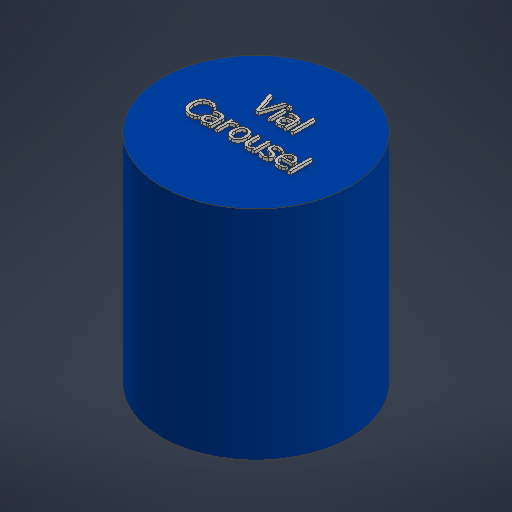
# Autodesk Inventor part: VialCarousel
Saved by Autodesk Inventor 2025.1 (Build 291241000, 241)
## iProperties
Created: 2024-10-04
Part Number: VialCarousel
Material: Generic
Document SubType Name: Modeling
Designer: jerem
Density: 1 g/cm^3
Appearance: Default
Author: jerem
Autodesk Inventor part; units mm, degrees
ref_plane "YZ Plane" through (0, 0, 0) normal (1, 0, 0) x (0, 1, 0)
ref_plane "XZ Plane" through (0, 0, 0) normal (0, 1, 0) x (-1, 0, 0)
ref_plane "XY Plane" through (0, 0, 0) normal (0, 0, 1) x (1, 0, 0)
sketch "Sketch1" plane through (0, 0, 0) normal (0, 1, 0) x (-1, 0, 0)
  circle A0 centre (0, 0) radius 65
  line L0 (0, 0) -> (0, -25) construction
  circle A1 centre (0, -25) radius 11.5 construction
  circle A2 centre (21.6506, -12.5) radius 11.5 construction
  circle A3 centre (21.6506, 12.5) radius 11.5 construction
  circle A4 centre (0, 25) radius 11.5 construction
  circle A5 centre (-21.6506, 12.5) radius 11.5 construction
  circle A6 centre (-21.6506, -12.5) radius 11.5 construction
  line L1 (0, 0) -> (-21.6506, 37.5) construction
  circle A7 centre (-21.6506, 37.5) radius 11.5 construction
  circle A8 centre (-43.3013, 0) radius 11.5 construction
  circle A9 centre (-21.6506, -37.5) radius 11.5 construction
  circle A10 centre (21.6506, -37.5) radius 11.5 construction
  circle A11 centre (43.3013, 0) radius 11.5 construction
  circle A12 centre (21.6506, 37.5) radius 11.5 construction
  circle A13 centre (0, 50) radius 11.5 construction
  circle A14 centre (-43.3013, 25) radius 11.5 construction
  circle A15 centre (-43.3013, -25) radius 11.5 construction
  circle A16 centre (0, -50) radius 11.5 construction
  circle A17 centre (43.3013, -25) radius 11.5 construction
  circle A18 centre (43.3013, 25) radius 11.5 construction
  dimension "d0" = 130
  dimension "d5" = 25
  dimension "d6" = 23
  dimension "d9" = 360
  dimension "d11" = 23
  dimension "d13" = 150
  dimension "d16" = 360
  dimension "d18" = 25
  dimension "d19" = 25
  dimension "d20" = 25
  dimension "d21" = 25
  dimension "d22" = 23
  dimension "d25" = 360
  constraints: 19 centre point, 4 end point, 3 coincident, 1 vertical, 39 other
  measures "d0" diameter of A0
  measures "d5" distance of L0.start L0.end
  measures "d6" diameter of A1
  measures "d11" diameter of A7
  measures "d13" angle of L1 L0
  measures "d18" distance of A12.centre A4.centre
  measures "d19" distance of A4.centre A3.centre
  measures "d20" distance of A4.centre A13.centre
  measures "d21" distance of A12.centre A13.centre
  measures "d22" diameter of A13
extrude "Extrusion1" add sketch "Sketch1" along normal blind 150
sketch "Sketch2" plane through (0, 150, 0) normal (0, 1, 0) x (1, 0, 0)
  line L0 (-43.9037, 26.5016) -> (43.579, 26.5016) construction
  line L1 (43.579, 26.5016) -> (43.579, 7.3742) construction
  line L2 (43.579, 7.3742) -> (-43.9037, 7.3742) construction
  line L3 (-43.9037, 7.3742) -> (-43.9037, 26.5016) construction
  line L4 (-4.0522, 25.8331) -> (-9.2183, 10.8331)
  line L5 (-9.2183, 10.8331) -> (-11.3698, 10.8331)
  line L6 (-11.3698, 10.8331) -> (-16.536, 25.8331)
  line L7 (-16.536, 25.8331) -> (-14.3966, 25.8331)
  line L8 (-14.3966, 25.8331) -> (-10.2394, 13.3736)
  line L9 (-10.2394, 13.3736) -> (-6.0821, 25.8331)
  line L10 (-6.0821, 25.8331) -> (-4.0522, 25.8331)
  line L11 (-0.8309, 10.8331) -> (-2.7272, 10.8331)
  line L12 (-2.7272, 10.8331) -> (-2.7272, 22.0891)
  line L13 (-2.7272, 22.0891) -> (-0.8309, 22.0891)
  line L14 (-0.8309, 22.0891) -> (-0.8309, 10.8331)
  line L15 (-0.6972, 23.9611) -> (-2.8488, 23.9611)
  line L16 (-2.8488, 23.9611) -> (-2.8488, 25.9303)
  line L17 (-2.8488, 25.9303) -> (-0.6972, 25.9303)
  line L18 (-0.6972, 25.9303) -> (-0.6972, 23.9611)
  spline S0 degree 2 poles (8.225, 12.0243) (7.994, 11.8541) (7.2161, 11.2463) (6.8514, 11.064) knots 0 0 0 1 2 2 2
  spline S1 degree 2 poles (6.8514, 11.064) (6.353, 10.7966) (5.417, 10.517) (4.5661, 10.517) knots 0 0 0 1 2 2 2
  spline S2 degree 2 poles (4.5661, 10.517) (3.8733, 10.517) (2.6213, 11.0397) (2.1472, 11.5138) knots 0 0 0 1 2 2 2
  spline S3 degree 2 poles (2.1472, 11.5138) (1.6974, 11.9757) (1.1504, 13.3371) (1.1504, 14.0908) knots 0 0 0 1 2 2 2
  spline S4 degree 2 poles (1.1504, 14.0908) (1.1504, 15.2577) (2.135, 16.9109) (3.2047, 17.3849) knots 0 0 0 1 2 2 2
  spline S5 degree 2 poles (3.2047, 17.3849) (4.1529, 17.8225) (6.7298, 18.1507) (8.225, 18.2358) knots 0 0 0 1 2 2 2
  line L19 (8.225, 18.2358) -> (8.225, 18.6005)
  spline S6 degree 2 poles (8.225, 18.6005) (8.225, 19.2569) (7.8238, 20.0713) (7.4592, 20.3023) knots 0 0 0 1 2 2 2
  spline S7 degree 2 poles (7.4592, 20.3023) (7.0945, 20.5332) (6.0491, 20.6791) (5.49, 20.6791) knots 0 0 0 1 2 2 2
  spline S8 degree 2 poles (5.49, 20.6791) (4.8336, 20.6791) (3.0589, 20.2901) (2.1715, 19.9133) knots 0 0 0 1 2 2 2
  line L20 (2.1715, 19.9133) -> (2.0621, 19.9133)
  line L21 (2.0621, 19.9133) -> (2.0621, 21.846)
  spline S9 degree 2 poles (2.0621, 21.846) (2.5848, 21.9919) (4.5418, 22.3566) (5.5021, 22.3566) knots 0 0 0 1 2 2 2
  spline S10 degree 2 poles (5.5021, 22.3566) (6.6691, 22.3566) (8.2614, 21.9919) (8.8935, 21.5178) knots 0 0 0 1 2 2 2
  spline S11 degree 2 poles (8.8935, 21.5178) (9.5135, 21.0559) (10.1213, 19.5851) (10.1213, 18.5275) knots 0 0 0 1 2 2 2
  line L22 (10.1213, 18.5275) -> (10.1213, 10.8331)
  line L23 (10.1213, 10.8331) -> (8.225, 10.8331)
  line L24 (8.225, 10.8331) -> (8.225, 12.0243)
  line L25 (8.225, 13.6045) -> (8.225, 16.7285)
  spline S12 degree 2 poles (8.225, 16.7285) (7.5443, 16.6677) (5.49, 16.4611) (4.8457, 16.2666) knots 0 0 0 1 2 2 2
  spline S13 degree 2 poles (4.8457, 16.2666) (4.0921, 16.0356) (3.1075, 15.0754) (3.1075, 14.2245) knots 0 0 0 1 2 2 2
  spline S14 degree 2 poles (3.1075, 14.2245) (3.1075, 13.252) (4.2015, 12.2674) (5.2469, 12.2674) knots 0 0 0 1 2 2 2
  spline S15 degree 2 poles (5.2469, 12.2674) (6.1342, 12.2674) (7.5929, 13.0332) (8.225, 13.6045) knots 0 0 0 1 2 2 2
  line L26 (14.7161, 10.8331) -> (12.8198, 10.8331)
  line L27 (12.8198, 10.8331) -> (12.8198, 26.5016)
  line L28 (12.8198, 26.5016) -> (14.7161, 26.5016)
  line L29 (14.7161, 26.5016) -> (14.7161, 10.8331)
  spline S16 degree 2 poles (-31.8459, -14.1315) (-33.3046, -14.1315) (-35.7722, -13.1469) (-36.6717, -12.1623) knots 0 0 0 1 2 2 2
  spline S17 degree 2 poles (-36.6717, -12.1623) (-37.5712, -11.1898) (-38.5558, -8.2725) (-38.5558, -6.3762) knots 0 0 0 1 2 2 2
  spline S18 degree 2 poles (-38.5558, -6.3762) (-38.5558, -4.4921) (-37.5955, -1.6963) (-36.6839, -0.6631) knots 0 0 0 1 2 2 2
  spline S19 degree 2 poles (-36.6839, -0.6631) (-35.7843, 0.3458) (-33.3289, 1.4034) (-31.8095, 1.4034) knots 0 0 0 1 2 2 2
  spline S20 degree 2 poles (-31.8095, 1.4034) (-31.0558, 1.4034) (-29.7309, 1.1846) (-29.1717, 1.0144) knots 0 0 0 1 2 2 2
  spline S21 degree 2 poles (-29.1717, 1.0144) (-28.6855, 0.8564) (-27.6766, 0.4066) (-27.1782, 0.1392) knots 0 0 0 1 2 2 2
  line L30 (-27.1782, 0.1392) -> (-27.1782, -2.2676)
  line L31 (-27.1782, -2.2676) -> (-27.3362, -2.2676)
  spline S22 degree 2 poles (-27.3362, -2.2676) (-27.6036, -2.0245) (-28.4302, -1.3438) (-29.0258, -1.0156) knots 0 0 0 1 2 2 2
  spline S23 degree 2 poles (-29.0258, -1.0156) (-29.5971, -0.6995) (-30.9464, -0.2984) (-31.8216, -0.2984) knots 0 0 0 1 2 2 2
  spline S24 degree 2 poles (-31.8216, -0.2984) (-32.7819, -0.2984) (-34.4958, -1.0885) (-35.1401, -1.8422) knots 0 0 0 1 2 2 2
  spline S25 degree 2 poles (-35.1401, -1.8422) (-35.7722, -2.608) (-36.4772, -4.9297) (-36.4772, -6.3762) knots 0 0 0 1 2 2 2
  spline S26 degree 2 poles (-36.4772, -6.3762) (-36.4772, -7.92) (-35.7357, -10.1444) (-35.0915, -10.9102) knots 0 0 0 1 2 2 2
  spline S27 degree 2 poles (-35.0915, -10.9102) (-34.4594, -11.6517) (-32.7698, -12.4054) (-31.8216, -12.4054) knots 0 0 0 1 2 2 2
  spline S28 degree 2 poles (-31.8216, -12.4054) (-30.9586, -12.4054) (-29.4877, -11.9799) (-28.9164, -11.6639) knots 0 0 0 1 2 2 2
  spline S29 degree 2 poles (-28.9164, -11.6639) (-28.3694, -11.3478) (-27.555, -10.6914) (-27.324, -10.4605) knots 0 0 0 1 2 2 2
  line L32 (-27.324, -10.4605) -> (-27.1782, -10.4605)
  line L33 (-27.1782, -10.4605) -> (-27.1782, -12.843)
  spline S30 degree 2 poles (-27.1782, -12.843) (-27.6766, -13.0739) (-28.5518, -13.4994) (-29.1717, -13.6939) knots 0 0 0 1 2 2 2
  spline S31 degree 2 poles (-29.1717, -13.6939) (-29.8281, -13.9127) (-30.9464, -14.1315) (-31.8459, -14.1315) knots 0 0 0 1 2 2 2
  spline S32 degree 2 poles (-19.192, -12.6728) (-19.4229, -12.843) (-20.2009, -13.4508) (-20.5655, -13.6331) knots 0 0 0 1 2 2 2
  spline S33 degree 2 poles (-20.5655, -13.6331) (-21.0639, -13.9005) (-21.9999, -14.1801) (-22.8508, -14.1801) knots 0 0 0 1 2 2 2
  spline S34 degree 2 poles (-22.8508, -14.1801) (-23.5437, -14.1801) (-24.7957, -13.6574) (-25.2698, -13.1833) knots 0 0 0 1 2 2 2
  spline S35 degree 2 poles (-25.2698, -13.1833) (-25.7195, -12.7214) (-26.2665, -11.36) (-26.2665, -10.6064) knots 0 0 0 1 2 2 2
  spline S36 degree 2 poles (-26.2665, -10.6064) (-26.2665, -9.4394) (-25.2819, -7.7863) (-24.2122, -7.3122) knots 0 0 0 1 2 2 2
  spline S37 degree 2 poles (-24.2122, -7.3122) (-23.2641, -6.8746) (-20.6871, -6.5464) (-19.192, -6.4613) knots 0 0 0 1 2 2 2
  line L34 (-19.192, -6.4613) -> (-19.192, -6.0966)
  spline S38 degree 2 poles (-19.192, -6.0966) (-19.192, -5.4402) (-19.5931, -4.6258) (-19.9578, -4.3948) knots 0 0 0 1 2 2 2
  spline S39 degree 2 poles (-19.9578, -4.3948) (-20.3224, -4.1639) (-21.3678, -4.018) (-21.927, -4.018) knots 0 0 0 1 2 2 2
  spline S40 degree 2 poles (-21.927, -4.018) (-22.5834, -4.018) (-24.3581, -4.407) (-25.2454, -4.7838) knots 0 0 0 1 2 2 2
  line L35 (-25.2454, -4.7838) -> (-25.3548, -4.7838)
  line L36 (-25.3548, -4.7838) -> (-25.3548, -2.8511)
  spline S41 degree 2 poles (-25.3548, -2.8511) (-24.8321, -2.7052) (-22.8751, -2.3405) (-21.9148, -2.3405) knots 0 0 0 1 2 2 2
  spline S42 degree 2 poles (-21.9148, -2.3405) (-20.7479, -2.3405) (-19.1555, -2.7052) (-18.5234, -3.1793) knots 0 0 0 1 2 2 2
  spline S43 degree 2 poles (-18.5234, -3.1793) (-17.9035, -3.6412) (-17.2957, -5.112) (-17.2957, -6.1696) knots 0 0 0 1 2 2 2
  line L37 (-17.2957, -6.1696) -> (-17.2957, -13.8641)
  line L38 (-17.2957, -13.8641) -> (-19.192, -13.8641)
  line L39 (-19.192, -13.8641) -> (-19.192, -12.6728)
  line L40 (-19.192, -11.0926) -> (-19.192, -7.9686)
  spline S44 degree 2 poles (-19.192, -7.9686) (-19.8727, -8.0294) (-21.927, -8.236) (-22.5712, -8.4305) knots 0 0 0 1 2 2 2
  spline S45 degree 2 poles (-22.5712, -8.4305) (-23.3249, -8.6615) (-24.3095, -9.6217) (-24.3095, -10.4726) knots 0 0 0 1 2 2 2
  spline S46 degree 2 poles (-24.3095, -10.4726) (-24.3095, -11.4451) (-23.2155, -12.4297) (-22.1701, -12.4297) knots 0 0 0 1 2 2 2
  spline S47 degree 2 poles (-22.1701, -12.4297) (-21.2827, -12.4297) (-19.824, -11.6639) (-19.192, -11.0926) knots 0 0 0 1 2 2 2
  line L41 (-8.6652, -4.638) -> (-8.7625, -4.638)
  spline S48 degree 2 poles (-8.7625, -4.638) (-8.9813, -4.5772) (-9.4553, -4.5529) (-9.7835, -4.5529) knots 0 0 0 1 2 2 2
  spline S49 degree 2 poles (-9.7835, -4.5529) (-10.5493, -4.5529) (-12.0566, -5.2214) (-12.7373, -5.8778) knots 0 0 0 1 2 2 2
  line L42 (-12.7373, -5.8778) -> (-12.7373, -13.8641)
  line L43 (-12.7373, -13.8641) -> (-14.6336, -13.8641)
  line L44 (-14.6336, -13.8641) -> (-14.6336, -2.608)
  line L45 (-14.6336, -2.608) -> (-12.7373, -2.608)
  line L46 (-12.7373, -2.608) -> (-12.7373, -4.2854)
  spline S50 degree 2 poles (-12.7373, -4.2854) (-11.7041, -3.3616) (-10.1604, -2.608) (-9.431, -2.608) knots 0 0 0 1 2 2 2
  spline S51 degree 2 poles (-9.431, -2.608) (-9.1393, -2.608) (-8.8475, -2.6323) (-8.6652, -2.6688) knots 0 0 0 1 2 2 2
  line L47 (-8.6652, -2.6688) -> (-8.6652, -4.638)
  spline S52 degree 2 poles (2.056, -8.236) (2.056, -11.0804) (-0.679, -14.1801) (-2.9642, -14.1801) knots 0 0 0 1 2 2 2
  spline S53 degree 2 poles (-2.9642, -14.1801) (-5.3103, -14.1801) (-7.9967, -10.9832) (-7.9967, -8.236) knots 0 0 0 1 2 2 2
  spline S54 degree 2 poles (-7.9967, -8.236) (-7.9967, -5.4159) (-5.2252, -2.2919) (-2.9642, -2.2919) knots 0 0 0 1 2 2 2
  spline S55 degree 2 poles (-2.9642, -2.2919) (-0.679, -2.2919) (2.056, -5.4038) (2.056, -8.236) knots 0 0 0 1 2 2 2
  spline S56 degree 2 poles (0.099, -8.236) (0.099, -6.048) (-1.4934, -3.9208) (-2.9642, -3.9208) knots 0 0 0 1 2 2 2
  spline S57 degree 2 poles (-2.9642, -3.9208) (-4.4351, -3.9208) (-6.0396, -6.048) (-6.0396, -8.236) knots 0 0 0 1 2 2 2
  spline S58 degree 2 poles (-6.0396, -8.236) (-6.0396, -10.3632) (-4.4351, -12.5512) (-2.9642, -12.5512) knots 0 0 0 1 2 2 2
  spline S59 degree 2 poles (-2.9642, -12.5512) (-1.5056, -12.5512) (0.099, -10.3997) (0.099, -8.236) knots 0 0 0 1 2 2 2
  line L48 (12.7529, -13.8641) -> (10.8567, -13.8641)
  line L49 (10.8567, -13.8641) -> (10.8567, -12.6242)
  spline S60 degree 2 poles (10.8567, -12.6242) (9.9815, -13.39) (8.4134, -14.1801) (7.4409, -14.1801) knots 0 0 0 1 2 2 2
  spline S61 degree 2 poles (7.4409, -14.1801) (6.7116, -14.1801) (5.411, -13.6939) (4.9369, -13.1712) knots 0 0 0 1 2 2 2
  spline S62 degree 2 poles (4.9369, -13.1712) (4.4507, -12.6485) (3.9158, -11.0561) (3.9158, -9.9135) knots 0 0 0 1 2 2 2
  line L50 (3.9158, -9.9135) -> (3.9158, -2.608)
  line L51 (3.9158, -2.608) -> (5.8121, -2.608)
  line L52 (5.8121, -2.608) -> (5.8121, -9.0261)
  spline S63 degree 2 poles (5.8121, -9.0261) (5.8121, -9.9256) (5.9458, -11.1047) (6.1768, -11.5423) knots 0 0 0 1 2 2 2
  spline S64 degree 2 poles (6.1768, -11.5423) (6.4077, -11.9799) (7.1978, -12.3811) (7.9393, -12.3811) knots 0 0 0 1 2 2 2
  spline S65 degree 2 poles (7.9393, -12.3811) (8.6322, -12.3811) (10.2003, -11.591) (10.8567, -11.0196) knots 0 0 0 1 2 2 2
  line L53 (10.8567, -11.0196) -> (10.8567, -2.608)
  line L54 (10.8567, -2.608) -> (12.7529, -2.608)
  line L55 (12.7529, -2.608) -> (12.7529, -13.8641)
  spline S66 degree 2 poles (18.539, -14.1315) (17.4085, -14.1315) (15.4515, -13.5237) (14.8072, -13.1833) knots 0 0 0 1 2 2 2
  line L56 (14.8072, -13.1833) -> (14.8072, -11.0561)
  line L57 (14.8072, -11.0561) -> (14.9045, -11.0561)
  spline S67 degree 2 poles (14.9045, -11.0561) (15.1476, -11.2506) (15.804, -11.7125) (16.351, -11.9678) knots 0 0 0 1 2 2 2
  spline S68 degree 2 poles (16.351, -11.9678) (16.8251, -12.1987) (17.992, -12.5391) (18.6119, -12.5391) knots 0 0 0 1 2 2 2
  spline S69 degree 2 poles (18.6119, -12.5391) (19.0617, -12.5391) (20.0949, -12.3324) (20.338, -12.1623) knots 0 0 0 1 2 2 2
  spline S70 degree 2 poles (20.338, -12.1623) (20.6905, -11.9313) (21.0066, -11.4086) (21.0066, -10.8738) knots 0 0 0 1 2 2 2
  spline S71 degree 2 poles (21.0066, -10.8738) (21.0066, -10.2052) (20.2773, -9.5123) (19.3413, -9.2814) knots 0 0 0 1 2 2 2
  spline S72 degree 2 poles (19.3413, -9.2814) (18.9766, -9.1963) (17.8097, -8.9532) (17.3113, -8.8195) knots 0 0 0 1 2 2 2
  spline S73 degree 2 poles (17.3113, -8.8195) (16.0228, -8.4427) (14.8559, -6.8867) (14.8559, -5.7806) knots 0 0 0 1 2 2 2
  spline S74 degree 2 poles (14.8559, -5.7806) (14.8559, -4.249) (17.1533, -2.3405) (19.0495, -2.3405) knots 0 0 0 1 2 2 2
  spline S75 degree 2 poles (19.0495, -2.3405) (19.9855, -2.3405) (21.8818, -2.8025) (22.526, -3.155) knots 0 0 0 1 2 2 2
  line L58 (22.526, -3.155) -> (22.526, -5.185)
  line L59 (22.526, -5.185) -> (22.4288, -5.185)
  spline S76 degree 2 poles (22.4288, -5.185) (21.6995, -4.6015) (19.9247, -3.9329) (19.0131, -3.9329) knots 0 0 0 1 2 2 2
  spline S77 degree 2 poles (19.0131, -3.9329) (18.0771, -3.9329) (16.7886, -4.723) (16.7886, -5.5132) knots 0 0 0 1 2 2 2
  spline S78 degree 2 poles (16.7886, -5.5132) (16.7886, -6.2303) (17.5544, -6.9232) (18.4053, -7.142) knots 0 0 0 1 2 2 2
  spline S79 degree 2 poles (18.4053, -7.142) (18.8186, -7.2514) (19.864, -7.4702) (20.4353, -7.6039) knots 0 0 0 1 2 2 2
  spline S80 degree 2 poles (20.4353, -7.6039) (21.6751, -7.92) (22.9393, -9.3665) (22.9393, -10.6185) knots 0 0 0 1 2 2 2
  spline S81 degree 2 poles (22.9393, -10.6185) (22.9393, -11.3478) (22.368, -12.6363) (21.8089, -13.1104) knots 0 0 0 1 2 2 2
  spline S82 degree 2 poles (21.8089, -13.1104) (21.2132, -13.6088) (19.6938, -14.1315) (18.539, -14.1315) knots 0 0 0 1 2 2 2
  spline S83 degree 2 poles (29.5884, -14.1193) (26.8899, -14.1193) (23.9239, -11.0926) (23.9239, -8.2968) knots 0 0 0 1 2 2 2
  spline S84 degree 2 poles (23.9239, -8.2968) (23.9239, -5.5496) (26.8048, -2.2919) (29.1265, -2.2919) knots 0 0 0 1 2 2 2
  spline S85 degree 2 poles (29.1265, -2.2919) (30.1719, -2.2919) (31.7886, -2.8997) (32.3842, -3.544) knots 0 0 0 1 2 2 2
  spline S86 degree 2 poles (32.3842, -3.544) (32.992, -4.1882) (33.6362, -6.048) (33.6362, -7.3973) knots 0 0 0 1 2 2 2
  line L60 (33.6362, -7.3973) -> (33.6362, -8.4305)
  line L61 (33.6362, -8.4305) -> (25.8445, -8.4305)
  spline S87 degree 2 poles (25.8445, -8.4305) (25.8445, -10.3876) (27.8137, -12.4662) (29.5641, -12.4662) knots 0 0 0 1 2 2 2
  spline S88 degree 2 poles (29.5641, -12.4662) (30.1841, -12.4662) (31.3875, -12.1866) (31.8737, -11.9678) knots 0 0 0 1 2 2 2
  spline S89 degree 2 poles (31.8737, -11.9678) (32.3842, -11.7247) (33.0892, -11.2992) (33.3202, -11.1047) knots 0 0 0 1 2 2 2
  line L62 (33.3202, -11.1047) -> (33.4296, -11.1047)
  line L63 (33.4296, -11.1047) -> (33.4296, -13.1712)
  spline S90 degree 2 poles (33.4296, -13.1712) (33.1014, -13.3049) (32.1046, -13.6939) (31.7157, -13.8033) knots 0 0 0 1 2 2 2
  spline S91 degree 2 poles (31.7157, -13.8033) (31.1687, -13.9613) (30.2691, -14.1193) (29.5884, -14.1193) knots 0 0 0 1 2 2 2
  spline S92 degree 2 poles (31.7886, -6.984) (31.7643, -6.2182) (31.4482, -5.0999) (31.1443, -4.723) knots 0 0 0 1 2 2 2
  spline S93 degree 2 poles (31.1443, -4.723) (30.8161, -4.2976) (29.7829, -3.8478) (29.0171, -3.8478) knots 0 0 0 1 2 2 2
  spline S94 degree 2 poles (29.0171, -3.8478) (28.2635, -3.8478) (27.2059, -4.2976) (26.7683, -4.7352) knots 0 0 0 1 2 2 2
  spline S95 degree 2 poles (26.7683, -4.7352) (26.3429, -5.185) (25.9053, -6.2668) (25.8445, -6.984) knots 0 0 0 1 2 2 2
  line L64 (25.8445, -6.984) -> (31.7886, -6.984)
  line L65 (37.4896, -13.8641) -> (35.5933, -13.8641)
  line L66 (35.5933, -13.8641) -> (35.5933, 1.8045)
  line L67 (35.5933, 1.8045) -> (37.4896, 1.8045)
  line L68 (37.4896, 1.8045) -> (37.4896, -13.8641)
  point P0 (0, 0)
  constraints: 2 other
extrude "Extrusion2" add sketch "Sketch2" along normal blind 2
equation "\"d11\" = d6"
equation "\"d21\" = d19"
equation "\"d22\" = d6"
body "Solid1"
